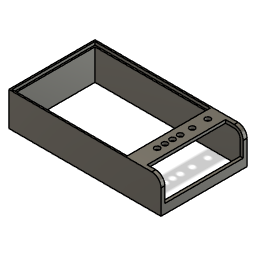
Tapa3_Inferior Final (Autodesk Fusion 360 design; units mm, degrees)
Autodesk Fusion 360 part; units mm, degrees
sketch "Boceto1" plane through (0, 0, 0) normal (0, 0, 1) x (1, 0, 0)
  line L0 (0, 0) -> (99, 0)
  line L1 (99, 0) -> (99, 22)
  line L2 (99, 22) -> (0, 22)
  line L3 (0, 22) -> (0, 0)
  dimension "d1" = 22
  dimension "d2" = 99
  constraint horizontal L0
  constraint vertical L1
  constraint horizontal L2
  constraint vertical L3
  constraint coincident L0.start L3.end
  measures "d1" distance of L0.end L1.end
  measures "d2" distance of L1.end L2.end
extrude "Extruir1" add sketch "Boceto1" along normal blind 56
shell "Vaciado1" thickness 2 removed faces 1 at (33, 0, 18.6667)
sketch "Boceto2" plane through (0, 22, 0) normal (0, 1, 0) x (-1, 0, 0)
  line L0 (-99, 0) -> (0, 0)
  line L1 (0, 0) -> (0, 56)
  line L2 (0, 56) -> (-99, 56)
  line L3 (-99, 56) -> (-99, 0)
  line L4 (-1, 1) -> (-76, 1)
  line L5 (-76, 1) -> (-76, 55)
  line L6 (-76, 55) -> (-1, 55)
  line L7 (-1, 55) -> (-1, 1)
  dimension "d6" = 1
  dimension "d7" = 1
  dimension "d8" = 1
  dimension "d9" = 75
  constraint horizontal L4
  constraint vertical L5
  constraint horizontal L6
  constraint vertical L7
  measures "d6" distance of L2 L6
  measures "d7" distance of L1 L7
  measures "d8" distance of L0 L4
  measures "d9" distance of L4.start L4.end
extrude "Extruir2" cut sketch "Boceto2" against normal blind 2 contours L4 L5 L6 L7
sketch "Boceto3" plane through (0, 22, 0) normal (0, 1, 0) x (-1, 0, 0)
  line L0 (-76, 1) -> (-76, 55)
  line L1 (-76, 55) -> (-1, 55)
  line L2 (-1, 55) -> (-1, 1)
  line L3 (-1, 1) -> (-76, 1)
  line L4 (-99, 0) -> (0, 0)
  line L5 (0, 0) -> (0, 56)
  line L6 (0, 56) -> (-99, 56)
  line L7 (-99, 56) -> (-99, 0)
  line L8 (-99, 2.5) -> (-87.5, 2.5)
  line L9 (-87.5, 2.5) -> (-87.5, 53.5)
  line L10 (-87.5, 53.5) -> (-99, 53.5)
  line L11 (-99, 53.5) -> (-99, 2.5)
  circle A0 centre (-81.4, 40.9) radius 1.75
  circle A1 centre (-81.4, 18.1) radius 1.75
  circle A2 centre (-81.4, 7.94) radius 1.75
  circle A3 centre (-81.4, 35.9) radius 1.75
  circle A4 centre (-81.4, 30.9) radius 1.75
  circle A5 centre (-81.4, 25.9) radius 1.75
  dimension "d12" = 2.5
  dimension "d13" = 2.5
  dimension "d14" = 11.5
  dimension "d29" = 0
  dimension "d30" = -15
  dimension "d31" = 6.1
  dimension "d32" = 3.5
  dimension "d33" = 3.5
  dimension "d34" = 3.5
  dimension "d35" = 10.16
  dimension "d36" = 12.6
  dimension "d37" = 7.8
  constraint horizontal L8
  constraint vertical L9
  constraint horizontal L10
  constraint vertical L11
  constraint coincident L7 L8.start
  constraint vertical A0.centre A1.centre
  constraint vertical A1.centre A2.centre
  measures "d12" distance of L6 L10
  measures "d13" distance of L4 L8
  measures "d14" distance of L9 L11
  measures "d31" distance of L9 A0.centre
  measures "d32" diameter of A0
  measures "d33" diameter of A1
  measures "d34" diameter of A2
  measures "d35" distance of A1.centre A2.centre
  measures "d36" distance of L10 A0.centre
  measures "d37" distance of A1.centre A5.centre
extrude "Extruir3" cut sketch "Boceto3" against normal blind 16 contours L7 L8 L9 L10 L11 | A0 | A1 | A2 | A3 | A4 | A5
fillet "Empalme1" radius 6 2 edges at (99, 22, 1.25) (99, 22, 54.75)
fillet "Empalme1" radius 4 2 edges at (97, 20, 2.25) (97, 20, 53.75)
equation "d35 = ( 4 * 2.54 ) * 1 mm"
